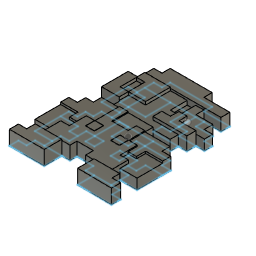
Mario (Autodesk Fusion 360 design; units mm, degrees)
Autodesk Fusion 360 part; units mm, degrees
note: some values were not read from the file. Chosen so that the rebuilt part matches the saved one: which bodies a step acts on.
sketch "Mario" plane through (0, 0, 0) normal (0, 0, 1) x (1, 0, 0)
  line L0 (-1.25, 3.3) -> (0.8, 3.3)
  line L1 (0.8, 3.3) -> (0.8, 2.9)
  line L2 (0.8, 2.9) -> (2.0624, 2.9)
  line L3 (2.0624, 2.9) -> (2.0624, 2.4642)
  line L4 (2.0624, 2.4642) -> (1.2358, 2.4642)
  line L5 (1.2358, 2.4642) -> (1.2358, 2.0717)
  line L6 (1.2358, 2.0717) -> (2.0624, 2.0717)
  line L7 (2.0624, 2.0717) -> (2.0624, 1.6465)
  line L8 (2.0624, 1.6465) -> (2.4727, 1.6465)
  line L9 (2.4727, 1.6465) -> (2.4727, 1.25)
  line L10 (2.4727, 1.25) -> (2.0624, 1.25)
  line L11 (2.0624, 1.25) -> (2.0624, 0.8)
  line L12 (2.0624, 0.8) -> (1.65, 0.8)
  line L13 (1.65, 0.8) -> (1.65, 0.4)
  line L14 (1.65, 0.4) -> (0.8199, 0.4)
  line L15 (0.8199, 0.4) -> (0.8199, 0)
  line L16 (0.8199, 0) -> (2.05, 0)
  line L17 (2.05, 0) -> (2.05, -0.4)
  line L18 (2.05, -0.4) -> (2.4822, -0.4)
  line L19 (2.4822, -0.4) -> (2.4822, -2.05)
  line L20 (2.4822, -2.05) -> (1.65, -2.05)
  line L21 (1.65, -2.05) -> (1.65, -2.4786)
  line L22 (1.65, -2.4786) -> (2.0661, -2.4786)
  line L23 (2.0661, -2.4786) -> (2.0661, -2.85)
  line L24 (2.0661, -2.85) -> (2.4826, -2.85)
  line L25 (2.4826, -2.85) -> (2.4826, -3.3)
  line L26 (2.4826, -3.3) -> (0.8126, -3.2792)
  line L27 (0.8126, -3.2792) -> (0.8126, -2.4786)
  line L28 (0.8126, -2.4786) -> (0.4, -2.4786)
  line L29 (0.4, -2.4786) -> (0.4, -2.1)
  line L30 (0.4, -2.1) -> (-0.4, -2.1)
  line L31 (-0.4, -2.1) -> (-0.4, -2.4416)
  line L32 (-0.7977, -2.4487) -> (-0.7977, -3.3)
  line L33 (-0.7977, -3.3) -> (-2.5, -3.3)
  line L34 (-2.5, -3.3) -> (-2.5, -2.8572)
  line L35 (-2.5, -2.8572) -> (-2.1, -2.8572)
  line L36 (-2.1, -2.8572) -> (-2.1, -2.4416)
  line L37 (-2.1, -2.4416) -> (-1.6558, -2.4416)
  line L38 (-1.6558, -2.4416) -> (-1.6558, -2.0544)
  line L39 (-1.6558, -2.0544) -> (-2.5, -2.0544)
  line L40 (-2.5, -2.0544) -> (-2.5, -0.4)
  line L41 (-2.5, -0.4) -> (-2.0779, -0.4)
  line L42 (-2.0779, -0.4) -> (-2.0779, 0)
  line L43 (-2.0779, 0) -> (-1.7, 0)
  line L44 (-1.7, 0) -> (-1.7, 0.4)
  line L45 (-1.7, 0.4) -> (-1.2, 0.4)
  line L46 (-1.2, 0.4) -> (-1.2, 0.8)
  line L47 (-1.2, 0.8) -> (-2.1, 0.8)
  line L48 (-2.1, 0.8) -> (-2.1, 2.1)
  line L49 (-2.1, 2.1) -> (-1.65, 2.1)
  line L50 (-1.65, 2.1) -> (-1.65, 2.9)
  line L51 (-1.65, 2.9) -> (-1.25, 2.9)
  line L52 (-1.25, 2.9) -> (-1.25, 3.3)
  line L53 (-1.6417, 2.0489) -> (-1.6417, 1.2477)
  line L54 (-1.6417, 1.2477) -> (-1.2372, 1.2477)
  line L55 (-1.2372, 1.2477) -> (-1.2372, 0.8)
  line L56 (-1.6417, 2.0489) -> (-1.2372, 2.0489)
  line L57 (-1.2372, 2.0489) -> (-1.2372, 1.2477)
  line L58 (-1.2372, 1.2477) -> (-0.4, 1.2477)
  line L59 (-0.4, 1.2477) -> (-0.4, 2.4612)
  line L60 (-0.4, 2.4612) -> (-1.65, 2.4612)
  line L61 (-0.4, 2.4612) -> (1.2358, 2.4642)
  line L62 (0.4179, 2.4627) -> (0.4179, 1.6424)
  line L63 (0.4179, 1.6424) -> (0.834, 1.6424)
  line L64 (0.834, 1.6424) -> (0.8325, 2.4634)
  line L65 (0.834, 1.6424) -> (1.2317, 1.6432)
  line L66 (1.2317, 1.6432) -> (1.2324, 1.2485)
  line L67 (1.2324, 1.2485) -> (2.0624, 1.25)
  line L68 (0.834, 1.6424) -> (0.8332, 2.0529)
  line L69 (0.4096, 1.2363) -> (0.8291, 1.2363)
  line L70 (0.8291, 1.2363) -> (0.834, 1.6424)
  line L71 (0.4096, 1.2363) -> (0.4096, 0.8)
  line L72 (0.4096, 0.8) -> (1.65, 0.8)
  line L73 (-0.83, 0.4033) -> (-0.83, -0.8)
  line L74 (-0.83, -0.8) -> (-1.2435, -0.8)
  line L75 (-1.2435, -0.8) -> (-1.2435, -1.6343)
  line L76 (-1.2435, -1.6343) -> (-1.6558, -1.6343)
  line L77 (-1.6558, -1.6343) -> (-1.6558, -2.0544)
  line L78 (-1.2435, -1.2171) -> (-1.6523, -1.2171)
  line L79 (-1.6523, -1.2171) -> (-1.6523, -0.8)
  line L80 (-1.6523, -0.8) -> (-2.5, -0.8)
  line L81 (-1.6558, -2.4416) -> (-0.7977, -2.4416)
  line L82 (-0.7977, -2.4416) -> (-0.7977, -2.4487)
  line L83 (-0.7977, -2.4416) -> (-0.4, -2.4416)
  line L84 (0.8126, -2.4786) -> (1.65, -2.4786)
  line L85 (1.65, -2.05) -> (1.65, -1.6365)
  line L86 (1.65, -1.6365) -> (1.2431, -1.6365)
  line L87 (1.2431, -1.6365) -> (1.2431, -0.8)
  line L88 (1.2431, -0.8) -> (0.8199, -0.8)
  line L89 (0.8199, 0) -> (0.8199, -0.8)
  line L90 (0.8199, 0) -> (0.4, 0)
  line L91 (0.4, 0) -> (0.4, -0.4)
  line L92 (0.4, -0.4) -> (-0.4, -0.4)
  line L93 (-0.4, -0.4) -> (-0.4, 0.4033)
  line L94 (-0.4, 0.4033) -> (-0.83, 0.4033)
  line L95 (-1.2, 0.4) -> (0.8199, 0.4)
  line L96 (-0.83, -0.8) -> (-0.4, -0.8)
  line L97 (-0.4, -0.8) -> (-0.4, -1.25)
  line L98 (-0.4, -1.25) -> (-0.83, -1.25)
  line L99 (-0.83, -1.25) -> (-0.83, -0.8)
  line L100 (0.8199, -0.8) -> (0.4, -0.8)
  line L101 (0.4, -0.8) -> (0.4, -1.25)
  line L102 (0.4, -1.25) -> (0.8199, -1.25)
  line L103 (0.8199, -1.25) -> (0.8199, -0.8)
  line L104 (1.2431, -1.25) -> (1.65, -1.25)
  line L105 (1.65, -1.25) -> (1.65, -0.8)
  line L106 (1.65, -0.8) -> (2.4822, -0.8)
  constraint horizontal L0
  constraint perpendicular L0 L1
  constraint perpendicular L1 L2
  constraint perpendicular L2 L3
  constraint perpendicular L3 L4
  constraint perpendicular L4 L5
  constraint perpendicular L5 L6
  constraint perpendicular L4 L7
  constraint perpendicular L7 L8
  constraint perpendicular L8 L9
  constraint perpendicular L7 L10
  constraint perpendicular L8 L11
  constraint perpendicular L11 L12
  constraint perpendicular L12 L13
  constraint perpendicular L11 L14
  constraint perpendicular L14 L15
  constraint perpendicular L15 L16
  constraint perpendicular L14 L17
  constraint perpendicular L17 L18
  constraint perpendicular L18 L19
  constraint perpendicular L19 L20
  constraint perpendicular L20 L21
  constraint perpendicular L21 L22
  constraint perpendicular L22 L23
  constraint perpendicular L23 L24
  constraint perpendicular L24 L25
  constraint perpendicular L24 L27
  constraint perpendicular L27 L28
  constraint perpendicular L28 L29
  constraint perpendicular L29 L30
  constraint perpendicular L30 L31
  constraint perpendicular L32 L33
  constraint perpendicular L33 L34
  constraint perpendicular L34 L35
  constraint perpendicular L35 L36
  constraint perpendicular L36 L37
  constraint perpendicular L37 L38
  constraint perpendicular L38 L39
  constraint perpendicular L39 L40
  constraint perpendicular L40 L41
  constraint perpendicular L41 L42
  constraint perpendicular L40 L43
  constraint perpendicular L43 L44
  constraint perpendicular L44 L45
  constraint perpendicular L45 L46
  constraint perpendicular L46 L47
  constraint perpendicular L47 L48
  constraint perpendicular L48 L49
  constraint perpendicular L47 L50
  constraint perpendicular L50 L51
  constraint perpendicular L0 L52
  constraint vertical L53
  constraint perpendicular L53 L54
  constraint coincident L47 L55.end
  constraint perpendicular L47 L55
  constraint perpendicular L53 L56
  constraint perpendicular L54 L57
  constraint perpendicular L57 L58
  constraint perpendicular L58 L59
  constraint coincident L50 L60.end
  constraint perpendicular L50 L60
  constraint midpoint L61 L62.start
  constraint perpendicular L62 L63
  constraint coincident L61 L64.end
  constraint perpendicular L61 L64
  constraint perpendicular L64 L65
  constraint perpendicular L65 L66
  constraint perpendicular L66 L67
  constraint perpendicular L65 L68
  constraint horizontal L69
  constraint perpendicular L69 L71
  constraint perpendicular L71 L72
  constraint vertical L73
  constraint perpendicular L73 L74
  constraint perpendicular L74 L75
  constraint perpendicular L75 L76
  constraint perpendicular L76 L77
  constraint midpoint L75 L78.start
  constraint perpendicular L75 L78
  constraint perpendicular L78 L79
  constraint coincident L40 L80.end
  constraint perpendicular L40 L80
  constraint perpendicular L38 L81
  constraint perpendicular L37 L82
  constraint perpendicular L32 L83
  constraint perpendicular L21 L84
  constraint perpendicular L20 L85
  constraint perpendicular L85 L86
  constraint perpendicular L86 L87
  constraint perpendicular L87 L88
  constraint perpendicular L88 L89
  constraint perpendicular L89 L90
  constraint perpendicular L90 L91
  constraint perpendicular L91 L92
  constraint perpendicular L90 L93
  constraint perpendicular L93 L94
  constraint perpendicular L15 L95
  constraint perpendicular L73 L96
  constraint perpendicular L96 L97
  constraint perpendicular L73 L98
  constraint perpendicular L96 L99
  constraint perpendicular L89 L100
  constraint perpendicular L100 L101
  constraint perpendicular L89 L102
  constraint perpendicular L100 L103
  constraint coincident L87 L104.start
  constraint perpendicular L87 L104
  constraint perpendicular L104 L105
  constraint coincident L19 L106.end
  constraint perpendicular L19 L106
extrude "Extrude1" add sketch "Mario" along normal blind 0.5 contours L53 L54 L56 L57 | L13 L14 L46 L47 L55 L58 L59 L61 L62 L63 L69 L70 L71 L72 L73 L93 L94 L95 | L5 L6 L7 L8 L9 L10 L61 L64 L65 L66 L67 L68 | L39 L40 L75 L76 L77 L78 L79 L80 | L19 L20 L85 L86 L87 L104 L105 L106 makes body 1 at (-1.2372, 1.7818, 0.1667) makes body 1 at (-0.1274, 1.7838, 0) makes body 1 at (0.9674, 2.0592, 0) makes body 2 at (2.2048, -1.3667, 0) makes body 3 at (-2.2186, -1.4962, 0)
extrude "Extrude2" add sketch "Mario" along normal blind 0.3 separate body contours L61 L62 L63 L64 L68 makes body 4
extrude "Extrude3" add sketch "Mario" along normal blind 0.6 separate body contours L0 L1 L2 L3 L4 L50 L51 L52 L60 L61 | L40 L41 L42 L43 L44 L45 L73 L74 L75 L78 L79 L80 L95 | L15 L90 L91 L92 L93 L95 | L16 L17 L18 L19 L87 L88 L89 L104 L105 L106 makes body 6 at (-0.1333, 0, 0) makes body 6 at (1.371, -0.2667, 0) makes body 5 at (-1.2578, -0.1333, 0) makes body 7 at (-0.2833, 3.0204, 0)
extrude "Extrude4" add sketch "Mario" along normal blind 0.65 separate body contours L47 L48 L49 L50 L55 L58 L59 L60 | L11 L12 L65 L66 L67 L69 L70 L71 L72 makes body 8 at (-0.6791, 1.9193, 0) makes body 9 at (1.5114, 0.8, 0.2167)
extrude "Extrude5" add sketch "Mario" along normal blind 0.65 separate body contours L21 L28 L29 L30 L31 L38 L73 L74 L75 L76 L77 L81 L83 L84 L85 L86 L87 L88 L89 L90 L91 L92 L93 L95 makes body 10
extrude "Extrude6" add sketch "Mario" along normal blind 0.7 separate body contours L32 L33 L34 L35 L36 L37 L81 L82 | L22 L23 L24 L25 L26 L27 L84 makes body 11 at (-1.2318, -2.8663, 0) makes body 12 at (1.2304, -2.8693, 0)
extrude "Extrude7" add sketch "Mario" along normal blind 0.66 contours L96 L97 L98 L99 | L100 L101 L102 L103 bodies 10 5 6
combine "Combine1" operation add target body 7 tool bodies 8 4 9 1 10 3 11 12 2
named bodies: "Mario"
